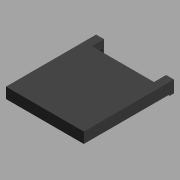
# Autodesk Inventor part: bin_lid
Saved by Autodesk Inventor 2019 (Build 230136000, 136)
## iProperties
Part Number: bin_lid
Material: Generic
Document SubType Name: Modeling
Designer: Javi
Appearance: Default
Author: Javi
Autodesk Inventor part; units mm, degrees
ref_plane "YZ Plane" through (0, 0, 0) normal (1, 0, 0) x (0, 1, 0)
ref_plane "XZ Plane" through (0, 0, 0) normal (0, 1, 0) x (-1, 0, 0)
ref_plane "XY Plane" through (0, 0, 0) normal (0, 0, 1) x (1, 0, 0)
sketch "Sketch1" plane through (0, 0, 0) normal (0, 1, 0) x (-1, 0, 0)
  line L0 (0, 0) -> (-436, 0)
  line L1 (-436, 0) -> (-436, -437)
  line L2 (-392, -437) -> (-44, -437)
  line L3 (0, -437) -> (0, 0)
  line L4 (0, -437) -> (0, -505)
  line L5 (0, -505) -> (-44, -505)
  line L6 (-44, -505) -> (-44, -437)
  line L7 (-436, -437) -> (-436, -505)
  line L8 (-436, -505) -> (-392, -505)
  line L9 (-392, -505) -> (-392, -437)
  dimension "d0" = 436
  dimension "d1" = 437
  dimension "d2" = 68
  dimension "d3" = 44
  dimension "d4" = 68
  dimension "d5" = 68
  dimension "d6" = 44
  dimension "d7" = 68
  constraints: 20 end point, 4 perpendicular, 2 parallel, 1 horizontal, 1 vertical
  measures "d0" distance of L3.start L1.end
  measures "d1" distance of L1.end L0.end
  measures "d2" distance of L3.start L4.end
  measures "d3" distance of L4.end L5.end
  measures "d4" distance of L2.end L5.end
  measures "d5" distance of L1.end L7.end
  measures "d6" distance of L7.end L8.end
  measures "d7" distance of L2.start L8.end
extrude "Extrusion1" add sketch "Sketch1" along normal blind 67
sketch "Sketch4" plane through (436, 0, 0) normal (1, 0, 0) x (0, 0, -1)
  line L0 (504.9333, 0) -> (480.9333, 0)
  line L1 (505, 0) -> (437, 0) projected
  line L2 (480.9333, 0) -> (473.8622, 7.0711)
  line L3 (473.8622, 7.0711) -> (0, 7.0711)
  line L4 (0, 0) -> (0, 67) projected
  line L5 (0, 7.0711) -> (0, 0)
  line L6 (0, 0) -> (480.9333, 0)
  dimension "d13" = 24
  dimension "d14" = 10
  dimension "d15" = 135
  constraints: 10 end point, 2 point on line, 1 parallel, 1 perpendicular, 1 vertical
  measures "d13" distance of L0.start L0.end
  measures "d14" distance of L0.end L2.end
  measures "d15" angle of L0 L2
extrude "Extrusion2" cut sketch "Sketch4" against normal through all
sketch "Sketch5" plane through (0, 0, 0) normal (0, -1, 0) x (1, 0, 0)
  line L0 (0, 0) -> (436, 0) projected
  line L1 (436, 0) -> (0, 0)
  line L2 (0, -505) -> (0, -480.9333) projected
  line L3 (0, 0) -> (0, -505)
  line L4 (44, -505) -> (0, -505) projected
  line L5 (0, -505) -> (44, -505)
  line L6 (44, -437) -> (44, -505) projected
  line L7 (44, -505) -> (44, -437)
  line L8 (392, -505) -> (392, -437) projected
  line L9 (44, -437) -> (392, -437)
  line L10 (392, -437) -> (392, -505)
  line L11 (436, -505) -> (392, -505) projected
  line L12 (392, -505) -> (436, -505)
  line L13 (436, 0) -> (436, -505) projected
  line L14 (436, -505) -> (436, 0)
  line L15 (396.4, -432.6) -> (39.6, -432.6)
  line L16 (39.6, -432.6) -> (39.6, -500.6)
  line L17 (39.6, -500.6) -> (4.4, -500.6)
  line L18 (4.4, -500.6) -> (4.4, -4.4)
  line L19 (4.4, -4.4) -> (431.6, -4.4)
  line L20 (431.6, -4.4) -> (431.6, -500.6)
  line L21 (431.6, -500.6) -> (396.4, -500.6)
  line L22 (396.4, -500.6) -> (396.4, -432.6)
  dimension "d18" = 4.4
  constraints: 32 end point, 8 perpendicular, 4 collinear, 7 other
  measures "d18" distance between parallel lines of L9 L15
extrude "Extrusion3" cut sketch "Sketch5" against normal blind 55 contours L15 L16 L17 L18 L19 L20 L21 L22
sketch "Sketch3" plane through (44, 0, -437) normal (1, 0, 0) x (0, 0, -1)
  circle A0 centre (54, 16) radius 7.5
  line L0 (0, 0) -> (0, 67) projected
  line L1 (0, 0) -> (68, 0) projected
  point P0 (-437, 0)
  dimension "d10" = 15
  dimension "d11" = 54
  dimension "d12" = 16
  constraints: 1 centre point
  measures "d10" diameter of A0
  measures "d11" distance from line of L0 A0.centre
  measures "d12" distance from line of L1 A0.centre
extrude "Extrusion4" cut sketch "Sketch3" along normal blind 367.5 and the other way blind 27.5
body "Solid1"
